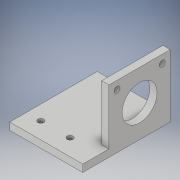
# Autodesk Inventor part: Backplate
Saved by Autodesk Inventor 2019 (Build 230136000, 136)
## iProperties
Created: 2021-06-02
Part Number: Backplate
Material: Generisch
Document SubType Name: Modeling
Designer: Bergi
Density: 1 g/cm^3
Appearance: Vorgabe
Author: Bergi
Autodesk Inventor part; units mm, degrees
ref_plane "YZ Plane" through (0, 0, 0) normal (1, 0, 0) x (0, 1, 0)
ref_plane "XZ Plane" through (0, 0, 0) normal (0, 1, 0) x (-1, 0, 0)
ref_plane "XY Plane" through (0, 0, 0) normal (0, 0, 1) x (1, 0, 0)
sketch "Skizze1" plane through (0, 0, 0) normal (0, 1, 0) x (-1, 0, 0)
  line L0 (-25, 30) -> (25, 30)
  line L1 (25, 30) -> (25, -30)
  line L2 (25, -30) -> (-25, -30)
  line L3 (-25, -30) -> (-25, 30)
  line L4 (-25, 30) -> (25, -30) construction
  line L5 (25, 30) -> (-25, -30) construction
  point P0 (0, 0)
  dimension "d0" = 50
  dimension "d1" = 60
  constraints: 12 end point, 2 midpoint, 2 parallel, 1 horizontal, 1 perpendicular
  measures "d0" distance of L1.end L2.end
  measures "d1" distance of L0.end L1.end
extrude "Extrusion1" add sketch "Skizze1" along normal blind 5
sketch "Skizze2" plane through (0, 5, 0) normal (0, 1, 0) x (1, 0, 0)
  line L0 (-25, -30) -> (25, -30) projected
  line L1 (25, -30) -> (25, 30) projected
  line L2 (25, 30) -> (-25, 30) projected
  line L3 (-25, 30) -> (-25, -30) projected
  line L4 (25, -30) -> (25, 30) projected
  line L5 (25, 30) -> (20, 30)
  line L6 (20, 30) -> (20, -12)
  line L7 (20, -12) -> (25, -12)
  line L8 (25, -12) -> (25, 30)
  point P0 (0, 0)
  dimension "d8" = 5
  dimension "d9" = 42
  constraints: 8 end point, 2 parallel, 1 horizontal, 1 perpendicular
  measures "d8" distance of L7.end L6.end
  measures "d9" distance of L6.end L5.end
extrude "Extrusion2" add sketch "Skizze2" along normal blind 38 contours L7 L6 L2 L1
sketch "Skizze3" plane through (25, 0, 30) normal (1, 0, 0) x (0, 0, -1)
  line L0 (60, 0) -> (0, 0) projected
  line L1 (60, 0) -> (60, 43) projected
  line L2 (18, 43) -> (60, 43) projected
  line L3 (18, 5) -> (18, 43) projected
  line L4 (0, 5) -> (18, 5) projected
  line L5 (0, 0) -> (0, 5) projected
  line L6 (39, -5.2039) -> (39, 72.0028) construction
  line L7 (23.5, 6.5) -> (54.5, 6.5) construction
  line L8 (54.5, 6.5) -> (54.5, 37.5) construction
  line L9 (54.5, 37.5) -> (23.5, 37.5) construction
  line L10 (23.5, 37.5) -> (23.5, 6.5) construction
  line L11 (23.5, 6.5) -> (54.5, 37.5) construction
  line L12 (54.5, 6.5) -> (23.5, 37.5) construction
  point P0 (30, 0)
  point P1 (39, 22)
  dimension "d10" = 21
  dimension "d11" = 17
  dimension "d19" = 31
  dimension "d20" = 31
  constraints: 14 end point, 2 coincident, 2 midpoint, 2 parallel, 1 horizontal, 1 perpendicular, 1 point on line, 1 vertical
  measures "d10" distance between parallel lines of L1 L6
  measures "d11" distance from line of L4 point (39, 22)
  measures "d19" distance of L9.end L8.end
  measures "d20" distance of L8.end L7.end
hole "Bohrung1" at (25, 22, -9) direction (-1, 0, 0) diameter 24 end through all
hole "Bohrung2" at (25, 37.5, 6.5) at (25, 37.5, -24.5) direction (-1, 0, 0) diameter 4 end through all
sketch "Skizze5" plane through (0, 0, 0) normal (0, -1, 0) x (1, 0, 0)
  line L0 (25, 30) -> (-25, 30) projected
  line L1 (-25, 30) -> (-25, -30) projected
  line L2 (-25, -30) -> (25, -30) projected
  line L3 (25, -30) -> (25, 30) projected
  line L4 (32.3204, 18.7) -> (-38.6965, 18.7) construction
  point P0 (0, 0)
  point P1 (-15, 18.7)
  point P2 (5, 18.7)
  dimension "d31" = 11.3
  dimension "d32" = 10
  dimension "d33" = 20
  constraints: 2 end point, 2 point on line, 1 horizontal
  measures "d31" distance between parallel lines of L0 L4
  measures "d32" distance from line of L1 point (-15, 18.7)
  measures "d33" distance of point (5, 18.7) point (-15, 18.7)
hole "Bohrung3" at (-15, 0, 18.7) at (5, 0, 18.7) direction (0, 1, 0) diameter 4 end through all counterbore diameter 8 counterbore depth 3
